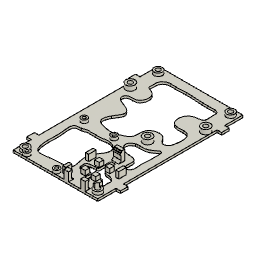
data-logger-inside-frame-504040 v42 (Autodesk Fusion 360 design; units mm, degrees)
Autodesk Fusion 360 part; units mm, degrees
sketch "Sketch1" plane through (0, 0, 0) normal (0, 0, 1) x (1, 0, 0)
  circle A0 centre (0, 0) radius 1.5
  circle A1 centre (0, 88) radius 1.5
  circle A2 centre (48, 0) radius 1.5
  circle A3 centre (48, 88) radius 1.5
  line L0 (-4, 92) -> (52, 92)
  line L1 (52, 92) -> (52, -4)
  line L2 (52, -4) -> (-4, -4)
  line L3 (-4, -4) -> (-4, 92)
  line L4 (-4, 80) -> (-7, 80)
  line L5 (-7, 80) -> (-7, 75)
  line L6 (-7, 75) -> (-4, 75)
  line L7 (-4, 75) -> (-4, 80)
  line L8 (52, 80) -> (55, 80)
  line L9 (55, 80) -> (55, 75)
  line L10 (55, 75) -> (52, 75)
  line L11 (52, 75) -> (52, 80)
  line L12 (-4, 13) -> (-7, 13)
  line L13 (-7, 13) -> (-7, 8)
  line L14 (-7, 8) -> (-4, 8)
  line L15 (-4, 8) -> (-4, 13)
  line L16 (52, 8) -> (55, 8)
  line L17 (55, 8) -> (55, 13)
  line L18 (55, 13) -> (52, 13)
  line L19 (52, 13) -> (52, 8)
  dimension "d1" = 3
  dimension "d2" = 3
  dimension "d3" = 88
  dimension "d4" = 3
  dimension "d5" = 48
  dimension "d6" = 3
  dimension "d7" = 56
  dimension "d8" = 96
  dimension "d9" = 4
  dimension "d10" = 4
  dimension "d11" = 3
  dimension "d12" = 5
  dimension "d13" = 3
  dimension "d14" = 5
  dimension "d15" = 3
  dimension "d16" = 5
  dimension "d17" = 3
  dimension "d18" = 5
  dimension "d19" = 12
  dimension "d20" = 12
  dimension "d21" = 12
  dimension "d22" = 12
  constraint coincident A0.centre origin
  constraint horizontal L0
  constraint vertical L1
  constraint horizontal L2
  constraint vertical L3
  constraint vertical A0.centre A1.centre
  constraint horizontal A0.centre A2.centre
  constraint horizontal A1.centre A3.centre
  constraint horizontal L4
  constraint vertical L5
  constraint horizontal L6
  constraint vertical L7
  constraint coincident L3 L4.start
  constraint horizontal L8
  constraint vertical L9
  constraint horizontal L10
  constraint vertical L11
  constraint coincident L1 L8.start
  constraint horizontal L12
  constraint vertical L13
  constraint horizontal L14
  constraint vertical L15
  constraint coincident L3 L12.start
  constraint horizontal L16
  constraint vertical L17
  constraint horizontal L18
  constraint vertical L19
  constraint coincident L1 L16.start
  measures "d1" diameter of A0
  measures "d2" diameter of A1
  measures "d3" distance of A0.centre A1.centre
  measures "d4" diameter of A2
  measures "d5" distance of A0.centre A2.centre
  measures "d6" diameter of A3
  measures "d7" distance of L0.start L0.end
  measures "d8" distance of L0.start L2.end
  measures "d9" distance of A1.centre L0
  measures "d10" distance of A1.centre L3
  measures "d11" distance of L4.start L4.end
  measures "d12" distance of L4.start L6.end
  measures "d13" distance of L8.start L8.end
  measures "d14" distance of L8.start L10.end
  measures "d15" distance of L12.start L12.end
  measures "d16" distance of L12.start L14.end
  measures "d17" distance of L16.start L16.end
  measures "d18" distance of L16.start L18.end
  measures "d19" distance of L0 L4
  measures "d20" distance of L2 L14
  measures "d21" distance of L2 L16
  measures "d22" distance of L0 L8
extrude "Extrude1" add sketch "Sketch1" along normal blind 1.5
sketch "Sketch2" plane through (0, 0, 1.5) normal (0, 0, 1) x (-1, 0, 0)
  circle A0 centre (-48, -88) radius 1.5
  circle A1 centre (-48, 0) radius 1.5
  circle A2 centre (0, 0) radius 1.5
  circle A3 centre (0, -88) radius 1.5
  line L0 (-52, -8) -> (-55, -8)
  line L1 (-55, -8) -> (-55, -13)
  line L2 (-55, -13) -> (-52, -13)
  line L3 (-52, -13) -> (-52, -75)
  line L4 (-52, -75) -> (-55, -75)
  line L5 (-55, -75) -> (-55, -80)
  line L6 (-55, -80) -> (-52, -80)
  line L7 (-52, -80) -> (-52, -92)
  line L8 (-52, -92) -> (4, -92)
  line L9 (4, -92) -> (4, -80)
  line L10 (4, -80) -> (7, -80)
  line L11 (7, -80) -> (7, -75)
  line L12 (7, -75) -> (4, -75)
  line L13 (4, -75) -> (4, -13)
  line L14 (4, -13) -> (7, -13)
  line L15 (7, -13) -> (7, -8)
  line L16 (7, -8) -> (4, -8)
  line L17 (4, -8) -> (4, 4)
  line L18 (4, 4) -> (-52, 4)
  line L19 (-52, 4) -> (-52, -8)
  line L20 (-27.6361, 2) -> (-45.6361, 2)
  line L21 (-45.6361, 2) -> (-45.6361, -24.25)
  line L22 (-45.6361, -24.25) -> (-27.6361, -24.25)
  line L23 (-27.6361, -24.25) -> (-27.6361, 2)
  line L24 (-29.6361, 2) -> (-32.6361, 2)
  line L25 (-32.6361, 2) -> (-32.6361, 4)
  line L26 (-32.6361, 4) -> (-29.6361, 4)
  line L27 (-29.6361, 4) -> (-29.6361, 2)
  line L28 (-40.6361, 2) -> (-43.6361, 2)
  line L29 (-43.6361, 2) -> (-43.6361, 4)
  line L30 (-43.6361, 4) -> (-40.6361, 4)
  line L31 (-40.6361, 4) -> (-40.6361, 2)
  line L32 (-34.1361, -24.25) -> (-39.1361, -24.25)
  line L33 (-39.1361, -24.25) -> (-39.1361, -26.75)
  line L34 (-39.1361, -26.75) -> (-34.1361, -26.75)
  line L35 (-34.1361, -26.75) -> (-34.1361, -24.25)
  line L36 (-27.6361, -19.25) -> (-25.6361, -19.25)
  line L37 (-25.6361, -19.25) -> (-25.6361, -14.25)
  line L38 (-25.6361, -14.25) -> (-27.6361, -14.25)
  line L39 (-27.6361, -14.25) -> (-27.6361, -19.25)
  line L40 (-45.6361, -19.25) -> (-47.6361, -19.25)
  line L41 (-47.6361, -19.25) -> (-47.6361, -14.25)
  line L42 (-47.6361, -14.25) -> (-45.6361, -14.25)
  line L43 (-45.6361, -14.25) -> (-45.6361, -19.25)
  line L44 (-27.6361, 0.8186) -> (-25.6361, 0.8186)
  line L45 (-25.6361, 0.8186) -> (-25.6361, -3.1814)
  line L46 (-25.6361, -3.1814) -> (-27.6361, -3.1814)
  line L47 (-27.6361, -3.1814) -> (-27.6361, 0.8186)
  line L48 (-45.6361, 0.5806) -> (-47.6361, 0.5806)
  line L49 (-47.6361, 0.5806) -> (-47.6361, -3.4194)
  line L50 (-47.6361, -3.4194) -> (-45.6361, -3.4194)
  line L51 (-45.6361, -3.4194) -> (-45.6361, 0.5806)
  line L52 (-0.7361, -38.1) -> (-24.9361, -38.1)
  line L53 (-24.9361, -38.1) -> (-24.9361, 4)
  line L54 (-24.9361, 4) -> (-0.7361, 4)
  line L55 (-0.7361, 4) -> (-0.7361, -38.1)
  circle A4 centre (-2.9611, -36.05) radius 1
  circle A5 centre (-2.9611, 1.95) radius 1
  circle A6 centre (-22.7111, -36.05) radius 1
  circle A7 centre (-22.7111, 1.95) radius 1
  circle A8 centre (-2.9611, -36.05) radius 2.05
  circle A9 centre (-22.7111, -36.05) radius 2.05
  circle A10 centre (-2.9611, 1.95) radius 2.05
  circle A11 centre (-22.7111, 1.95) radius 2.05
  circle A12 centre (0, 0) radius 2.75
  circle A13 centre (-48, 0) radius 2.75
  circle A14 centre (0, -88) radius 2.75
  circle A15 centre (-48, -88) radius 2.75
  circle A16 centre (1, -70.5) radius 3
  circle A17 centre (-49, -70.5) radius 3
  circle A18 centre (-35.5, -45.5) radius 3
  line L56 (-51.3515, -29.8744) -> (-23.0253, -29.8744)
  line L57 (-23.0253, -29.8744) -> (-23.0253, 4)
  line L58 (-23.0253, 4) -> (-51.3515, 4)
  line L59 (-51.3515, 4) -> (-51.3515, -29.8744)
  dimension "d25" = 18
  dimension "d26" = 26.25
  dimension "d27" = 2
  dimension "d28" = 3
  dimension "d29" = 3
  dimension "d30" = 2
  dimension "d31" = 2
  dimension "d32" = 5
  dimension "d33" = 2.5
  dimension "d34" = 6.5
  dimension "d35" = 2
  dimension "d36" = 5
  dimension "d37" = 2
  dimension "d38" = 5
  dimension "d39" = 5
  dimension "d40" = 5
  dimension "d41" = 2
  dimension "d42" = 4
  dimension "d43" = 2
  dimension "d44" = 4
  dimension "d45" = 42.1
  dimension "d46" = 24.2
  dimension "d47" = 2
  dimension "d48" = 2
  dimension "d49" = 2
  dimension "d50" = 2
  dimension "d51" = 19.75
  dimension "d52" = 38
  dimension "d53" = 2.05
  dimension "d54" = 2.225
  dimension "d57" = 0.7
  dimension "d76" = 5.5
  dimension "d77" = 5.5
  dimension "d78" = 5.5
  dimension "d79" = 5.5
  dimension "d141" = 6
  dimension "d142" = 6
  dimension "d143" = 6
  dimension "d144" = 50
  dimension "d145" = 25
  dimension "d146" = 13.5
  dimension "d149" = 21.5
  dimension "d150" = 7.4
  constraint horizontal L20
  constraint vertical L21
  constraint horizontal L22
  constraint vertical L23
  constraint horizontal L24
  constraint vertical L25
  constraint horizontal L26
  constraint vertical L27
  constraint coincident L20 L24.start
  constraint horizontal L28
  constraint vertical L29
  constraint horizontal L30
  constraint vertical L31
  constraint coincident L20 L28.start
  constraint horizontal L32
  constraint vertical L33
  constraint horizontal L34
  constraint vertical L35
  constraint coincident L22 L32.start
  constraint horizontal L36
  constraint vertical L37
  constraint horizontal L38
  constraint vertical L39
  constraint coincident L23 L36.start
  constraint horizontal L40
  constraint vertical L41
  constraint horizontal L42
  constraint vertical L43
  constraint coincident L21 L40.start
  constraint horizontal L44
  constraint vertical L45
  constraint horizontal L46
  constraint vertical L47
  constraint coincident L23 L44.start
  constraint horizontal L48
  constraint vertical L49
  constraint horizontal L50
  constraint vertical L51
  constraint coincident L21 L48.start
  constraint horizontal L52
  constraint vertical L53
  constraint horizontal L54
  constraint vertical L55
  constraint coincident L18 L54.end
  constraint horizontal A4.centre A6.centre
  constraint vertical A4.centre A5.centre
  constraint vertical A6.centre A7.centre
  constraint horizontal A5.centre A7.centre
  constraint concentric A4 A8
  constraint tangent L52 A8
  constraint concentric A6 A9
  constraint tangent L52 A9
  constraint concentric A5 A10
  constraint tangent L54 A10
  constraint concentric A7 A11
  constraint tangent L54 A11
  constraint coincident A2.centre A12.centre
  constraint concentric A1 A13
  constraint concentric A3 A14
  constraint concentric A0 A15
  constraint horizontal A16.centre A17.centre
  constraint tangent L3 A17
  constraint horizontal L56
  constraint vertical L57
  constraint horizontal L58
  constraint vertical L59
  constraint coincident L54 L57.end
  measures "d25" distance of L20.start L20.end
  measures "d26" distance of L20.start L22.end
  measures "d27" distance of L18 L20
  measures "d28" distance of L24.start L24.end
  measures "d29" distance of L28.start L28.end
  measures "d30" distance of L23 L26.end
  measures "d31" distance of L21 L29
  measures "d32" distance of L32.start L32.end
  measures "d33" distance of L32.start L34.end
  measures "d34" distance of L21 L33
  measures "d35" distance of L36.start L36.end
  measures "d36" distance of L36.start L38.end
  measures "d37" distance of L40.start L40.end
  measures "d38" distance of L40.start L42.end
  measures "d39" distance of L22 L36
  measures "d40" distance of L22 L40
  measures "d41" distance of L44.start L44.end
  measures "d42" distance of L44.start L46.end
  measures "d43" distance of L48.start L48.end
  measures "d44" distance of L48.start L50.end
  measures "d45" distance of L52.start L54.end
  measures "d46" distance of L52.start L52.end
  measures "d47" diameter of A4
  measures "d48" diameter of A5
  measures "d49" diameter of A6
  measures "d50" diameter of A7
  measures "d51" distance of A4.centre A6.centre
  measures "d52" distance of A4.centre A5.centre
  measures "d53" distance of L52 A4.centre
  measures "d54" distance of L55 A4.centre
  measures "d57" distance of L37 L53
  measures "d76" diameter of A12
  measures "d77" diameter of A13
  measures "d78" diameter of A14
  measures "d79" diameter of A15
  measures "d141" diameter of A16
  measures "d142" diameter of A17
  measures "d143" diameter of A18
  measures "d144" distance of A16.centre A17.centre
  measures "d145" vertical distance of A16.centre A18.centre
  measures "d146" horizontal distance of A17.centre A18.centre
  measures "d149" distance of L8 A16.centre
  measures "d150" distance of L52 A18.centre
extrude "Extrude21" add sketch "Sketch2" along normal blind 3 contours A17 | A16 | A18
extrude "Extrude6" add sketch "Sketch2" along normal blind 2 contours A1 L21 L48 L49 A13 | L21 L51 A13 | A2 L55 A10 A12 | A2 L55 A10 A12 | A2 L55 A12 | A14 | A15
extrude "Extrude3" cut sketch "Sketch2" against normal blind 3 contours A7 L57 | A7 L57 | A5 A12 | A5 A12 | A4 | A6
extrude "Extrude2" add sketch "Sketch2" along normal blind 2 contours A9 | A8 | A7 A11 L57 | A7 A11 L57 | A5 A10 A12 | A2 A5 A10 A12 | A2 A10
sketch "Sketch3" plane through (0, 0, 1.5) normal (0, 0, 1) x (-1, 0, 0)
  line L0 (-41.6361, -5) -> (-38.6361, -5)
  line L1 (-38.6361, -5) -> (-38.6361, -8)
  line L2 (-38.6361, -8) -> (-41.6361, -8)
  line L3 (-41.6361, -8) -> (-41.6361, -5)
  line L4 (-34.6361, -5) -> (-31.6361, -5)
  line L5 (-31.6361, -5) -> (-31.6361, -8)
  line L6 (-31.6361, -8) -> (-34.6361, -8)
  line L7 (-34.6361, -8) -> (-34.6361, -5)
  line L8 (-41.6361, -14.25) -> (-38.6361, -14.25)
  line L9 (-38.6361, -14.25) -> (-38.6361, -17.25)
  line L10 (-38.6361, -17.25) -> (-41.6361, -17.25)
  line L11 (-41.6361, -17.25) -> (-41.6361, -14.25)
  line L12 (-31.6361, -14.25) -> (-34.6361, -14.25)
  line L13 (-34.6361, -14.25) -> (-34.6361, -17.25)
  line L14 (-34.6361, -17.25) -> (-31.6361, -17.25)
  line L15 (-31.6361, -17.25) -> (-31.6361, -14.25)
  line L16 (-27.6361, 2) -> (-45.6361, 2)
  line L17 (-45.6361, 2) -> (-45.6361, -24.25)
  line L18 (-45.6361, -24.25) -> (-27.6361, -24.25)
  line L19 (-27.6361, -24.25) -> (-27.6361, 2)
  dimension "d60" = 3
  dimension "d61" = 3
  dimension "d62" = 3
  dimension "d63" = 3
  dimension "d64" = 3
  dimension "d65" = 3
  dimension "d66" = 3
  dimension "d67" = 3
  dimension "d68" = 7
  dimension "d69" = 4
  dimension "d70" = 7
  dimension "d71" = 4
  constraint horizontal L0
  constraint vertical L1
  constraint horizontal L2
  constraint vertical L3
  constraint horizontal L4
  constraint vertical L5
  constraint horizontal L6
  constraint vertical L7
  constraint horizontal L8
  constraint vertical L9
  constraint horizontal L10
  constraint vertical L11
  constraint horizontal L12
  constraint vertical L13
  constraint horizontal L14
  constraint vertical L15
  constraint horizontal L0.start L4.start
  constraint vertical L0.start L8.start
  constraint horizontal L8.start L12.end
  constraint vertical L4.start L12.end
  measures "d60" distance of L0.start L0.end
  measures "d61" distance of L0.start L2.end
  measures "d62" distance of L4.start L4.end
  measures "d63" distance of L4.start L6.end
  measures "d64" distance of L8.start L8.end
  measures "d65" distance of L8.start L10.end
  measures "d66" distance of L12.start L12.end
  measures "d67" distance of L12.start L14.end
  measures "d68" distance of L0 L16
  measures "d69" distance of L3 L17
  measures "d70" distance of L10 L18
  measures "d71" distance of L5 L19
extrude "Extrude4" add sketch "Sketch3" along normal blind 3 contours L0 L1 L2 L3 | L4 L5 L6 L7 | L8 L9 L10 L11 | L12 L13 L14 L15
extrude "Extrude5" add sketch "Sketch2" along normal blind 4.2 contours A1 L21 L48 L49 L51 A13 | L21 L49 L50 L51 A13 | L18 L20 L28 L29 L30 L31 L58 | L21 L40 L41 L42 L43 | L18 L20 L24 L25 L26 L27 L58 | L22 L32 L33 L34 L35 | L23 L44 L45 L46 L47 | L23 L36 L37 L38 L39
sketch "Sketch4" plane through (0, 0, 5.7) normal (0, 0, 1) x (-1, 0, 0)
  line L0 (-34.1361, -26.75) -> (-34.1361, -24.25)
  line L1 (-34.1361, -24.25) -> (-39.1361, -24.25)
  line L2 (-39.1361, -24.25) -> (-39.1361, -26.75)
  line L3 (-39.1361, -26.75) -> (-34.1361, -26.75)
  line L4 (-34.1361, -26.75) -> (-39.1361, -26.75)
  line L5 (-39.1361, -26.75) -> (-39.1361, -23.75)
  line L6 (-39.1361, -23.75) -> (-34.1361, -23.75)
  line L7 (-34.1361, -23.75) -> (-34.1361, -26.75)
  dimension "d82" = 5
  dimension "d83" = 3
  constraint horizontal L4
  constraint vertical L5
  constraint horizontal L6
  constraint vertical L7
  constraint coincident L0.start L3.end
  measures "d82" distance of L0.start L2.end
  measures "d83" distance of L0.start L6.end
extrude "Extrude7" add sketch "Sketch4" along normal blind 1.5
sketch "Sketch5" plane through (0, 0, 5.7) normal (0, 0, 1) x (-1, 0, 0)
  line L0 (-27.6361, -14.25) -> (-27.6361, -19.25)
  line L1 (-27.6361, -19.25) -> (-25.6361, -19.25)
  line L2 (-25.6361, -19.25) -> (-25.6361, -14.25)
  line L3 (-25.6361, -14.25) -> (-27.6361, -14.25)
  line L4 (-25.6361, -19.25) -> (-28.1361, -19.25)
  line L5 (-28.1361, -19.25) -> (-28.1361, -14.25)
  line L6 (-28.1361, -14.25) -> (-25.6361, -14.25)
  line L7 (-25.6361, -14.25) -> (-25.6361, -19.25)
  dimension "d86" = 2.5
  dimension "d87" = 5
  constraint horizontal L4
  constraint vertical L5
  constraint horizontal L6
  constraint vertical L7
  constraint coincident L1.end L2.start
  measures "d86" distance of L1.end L4.end
  measures "d87" distance of L1.end L2.end
sketch "Sketch9" plane through (0, 0, 5.7) normal (0, 0, 1) x (-1, 0, 0)
  line L0 (-29.6361, 4) -> (-32.6361, 4)
  line L1 (-32.6361, 4) -> (-32.6361, 2)
  line L2 (-32.6361, 2) -> (-29.6361, 2)
  line L3 (-29.6361, 2) -> (-29.6361, 4)
  line L4 (-29.6361, 4) -> (-32.6361, 4)
  line L5 (-32.6361, 4) -> (-32.6361, 1.5)
  line L6 (-32.6361, 1.5) -> (-29.6361, 1.5)
  line L7 (-29.6361, 1.5) -> (-29.6361, 4)
  dimension "d103" = 2.5
  constraint horizontal L4
  constraint vertical L5
  constraint horizontal L6
  constraint vertical L7
  constraint coincident L0.start L3.end
  constraint coincident L5.end L6.start
  measures "d103" distance of L0.start L6.end
extrude "Extrude12" add sketch "Sketch9" along normal blind 1.5
sketch "Sketch10" plane through (0, 0, 5.7) normal (0, 0, 1) x (-1, 0, 0)
  line L0 (-40.6361, 4) -> (-43.6361, 4)
  line L1 (-43.6361, 4) -> (-43.6361, 2)
  line L2 (-43.6361, 2) -> (-40.6361, 2)
  line L3 (-40.6361, 2) -> (-40.6361, 4)
  line L4 (-40.6361, 4) -> (-43.6361, 4)
  line L5 (-43.6361, 4) -> (-43.6361, 1.5)
  line L6 (-43.6361, 1.5) -> (-40.6361, 1.5)
  line L7 (-40.6361, 1.5) -> (-40.6361, 4)
  dimension "d167" = 2.5
  constraint horizontal L4
  constraint vertical L5
  constraint horizontal L6
  constraint vertical L7
  constraint coincident L0.start L3.end
  measures "d167" distance of L0.start L6.end
extrude "Extrude27" add sketch "Sketch10" along normal blind 1.5
chamfer "Chamfer4" distance 0.5 angle 45 3 edges at (42.1361, -1.5, 5.7) (31.1361, -1.5, 5.7) (36.6361, 23.75, 5.7) measured on face at (42.6361, -1.5, 6.2) measured on face at (31.6361, -1.5, 6.2) measured on face at (37.4695, 23.9167, 5.7)
thread "Thread2" [suppressed]
sketch "Sketch17" plane through (0, 0, 4.5) normal (0, 0, 1) x (-1, 0, 0)
  circle A0 centre (1, -70.5) radius 3
  circle A1 centre (1, -70.5) radius 1.5
  dimension "d153" = 3
  constraint concentric A0 A1
  measures "d153" diameter of A1
extrude "Extrude22" cut sketch "Sketch17" against normal blind 7 contours A1
sketch "Sketch18" plane through (0, 0, 4.5) normal (0, 0, 1) x (-1, 0, 0)
  circle A0 centre (-49, -70.5) radius 3
  circle A1 centre (-49, -70.5) radius 1.5
  dimension "d156" = 3
  constraint concentric A0 A1
  measures "d156" diameter of A1
extrude "Extrude23" cut sketch "Sketch18" against normal blind 7 contours A1
sketch "Sketch19" plane through (0, 0, 4.5) normal (0, 0, 1) x (-1, 0, 0)
  circle A0 centre (-35.5, -45.5) radius 3
  circle A1 centre (-35.5, -45.5) radius 1.5
  dimension "d159" = 3
  constraint concentric A0 A1
  measures "d159" diameter of A1
extrude "Extrude24" cut sketch "Sketch19" against normal blind 7 contours A1
sketch "Sketch20" plane through (0, 0, 1.5) normal (0, 0, 1) x (-1, 0, 0)
  line L0 (-34.1361, -26.75) -> (-39.1361, -26.75)
  line L1 (-39.1361, -26.75) -> (-39.1361, -24.25)
  line L2 (-39.1361, -24.25) -> (-34.1361, -24.25)
  line L3 (-34.1361, -24.25) -> (-34.1361, -26.75)
  line L4 (-43.6361, 2) -> (-43.6361, 4)
  line L5 (-43.6361, 4) -> (-52, 4)
  line L6 (-52, 4) -> (-52, -8)
  line L7 (-52, -13) -> (-52, -70.5)
  circle A0 centre (-49, -70.5) radius 3
  line L8 (-52, -80) -> (-52, -92)
  line L9 (-52, -92) -> (4, -92)
  line L10 (4, -92) -> (4, -80)
  line L11 (4, -75) -> (4, -70.5)
  circle A1 centre (1, -70.5) radius 3
  line L12 (4, -8) -> (4, 4)
  line L13 (4, 4) -> (-2.9611, 4)
  arc A2 (-1.004, 2.5602) -> (-2.9611, 4) centre (-2.9611, 1.95) ccw
  arc A3 (-2.7486, -0.0889) -> (-1.004, 2.5602) centre (0, 0) ccw
  arc A4 (-2.9611, 4) -> (-2.7486, -0.0889) centre (-2.9611, 1.95) ccw
  line L14 (-2.9611, 4) -> (-22.7111, 4)
  circle A5 centre (-22.7111, 1.95) radius 2.05
  line L15 (-22.7111, 4) -> (-29.6361, 4)
  line L16 (-29.6361, 4) -> (-29.6361, 2)
  line L17 (-29.6361, 2) -> (-32.6361, 2)
  line L18 (-32.6361, 2) -> (-32.6361, 4)
  line L19 (-32.6361, 4) -> (-40.6361, 4)
  line L20 (-40.6361, 4) -> (-40.6361, 2)
  line L21 (-40.6361, 2) -> (-43.6361, 2)
  line L22 (-45.6361, -14.25) -> (-45.6361, -19.25)
  line L23 (-45.6361, -19.25) -> (-47.6361, -19.25)
  line L24 (-47.6361, -19.25) -> (-47.6361, -14.25)
  line L25 (-47.6361, -14.25) -> (-45.6361, -14.25)
  line L26 (-27.6361, -14.25) -> (-25.6361, -14.25)
  line L27 (-25.6361, -14.25) -> (-25.6361, -19.25)
  line L28 (-25.6361, -19.25) -> (-27.6361, -19.25)
  line L29 (-27.6361, -19.25) -> (-27.6361, -14.25)
  line L30 (-47.6361, -3.4194) -> (-47.6361, -2.7258)
  arc A6 (-45.6361, -1.4052) -> (-47.6361, -2.7258) centre (-48, 0) ccw
  line L31 (-45.6361, -1.4052) -> (-45.6361, -3.4194)
  line L32 (-45.6361, -3.4194) -> (-47.6361, -3.4194)
  line L33 (-27.6361, -3.1814) -> (-27.6361, 0.8186)
  line L34 (-27.6361, 0.8186) -> (-25.6361, 0.8186)
  line L35 (-25.6361, 0.8186) -> (-25.6361, -3.1814)
  line L36 (-25.6361, -3.1814) -> (-27.6361, -3.1814)
  line L37 (-31.6361, -17.25) -> (-34.6361, -17.25)
  line L38 (-34.6361, -17.25) -> (-34.6361, -14.25)
  line L39 (-34.6361, -14.25) -> (-31.6361, -14.25)
  line L40 (-31.6361, -14.25) -> (-31.6361, -17.25)
  line L41 (-41.6361, -8) -> (-41.6361, -5)
  line L42 (-41.6361, -5) -> (-38.6361, -5)
  line L43 (-38.6361, -5) -> (-38.6361, -8)
  line L44 (-38.6361, -8) -> (-41.6361, -8)
  line L45 (-41.6361, -17.25) -> (-41.6361, -14.25)
  line L46 (-41.6361, -14.25) -> (-38.6361, -14.25)
  line L47 (-38.6361, -14.25) -> (-38.6361, -17.25)
  line L48 (-38.6361, -17.25) -> (-41.6361, -17.25)
  line L49 (-34.6361, -8) -> (-34.6361, -5)
  line L50 (-34.6361, -5) -> (-31.6361, -5)
  line L51 (-31.6361, -5) -> (-31.6361, -8)
  line L52 (-31.6361, -8) -> (-34.6361, -8)
  circle A7 centre (-48, -88) radius 2.75
  circle A8 centre (-35.5, -45.5) radius 3
  circle A9 centre (0, -88) radius 2.75
  circle A10 centre (-22.7111, -36.05) radius 2.05
  circle A11 centre (-2.9611, -36.05) radius 2.05
  spline S0 degree 5 poles (-6, -31) (-6.2089, -31.0339) (-6.6159, -31.1153) (-7.1879, -31.2803) (-7.8646, -31.5655) (-8.5955, -31.9042) (-9.2655, -32.0974) (-9.9265, -32.1123) (-10.6133, -32.0311) (-11.3495, -31.9614) (-12.1493, -31.9557) (-13.0188, -31.9882) (-13.9539, -32.011) (-14.94, -31.9882) (-15.95, -31.9402) (-16.9546, -31.9166) (-17.934, -31.968) (-18.8872, -32.1183) (-19.8451, -32.3353) (-20.8523, -32.5494) (-21.9471, -32.6766) (-23.144, -32.6391) (-24.4104, -32.3902) (-25.6743, -31.9152) (-26.8437, -31.223) (-27.8225, -30.3407) (-28.5269, -29.307) (-28.9041, -28.1664) (-28.9362, -26.9626) (-28.6372, -25.7333) (-28.0528, -24.5033) (-27.2584, -23.2789) (-26.3589, -22.0419) (-25.4727, -20.7585) (-24.7153, -19.3908) (-24.1834, -17.9066) (-23.9382, -16.2903) (-23.99, -14.5526) (-24.2794, -12.7428) (-24.6941, -10.938) (-25.0935, -9.2281) (-25.3296, -7.7021) (-25.2707, -6.4341) (-24.8214, -5.47) (-23.9499, -4.8103) (-22.6896, -4.4111) (-21.1163, -4.2024) (-19.3322, -4.1019) (-17.4465, -4.0304) (-15.559, -3.9263) (-13.739, -3.7625) (-12.0271, -3.5446) (-10.4431, -3.3032) (-8.9917, -3.0875) (-7.6698, -2.9594) (-6.4717, -2.9865) (-5.3975, -3.2362) (-4.4546, -3.7684) (-3.653, -4.6251) (-3.0024, -5.8213) (-2.5079, -7.3358) (-2.1664, -9.1008) (-1.9661, -11.0201) (-1.886, -12.9914) (-1.8959, -14.9248) (-1.9546, -16.7676) (-2.0136, -18.5154) (-2.0062, -20.2553) (-1.8716, -22.1348) (-1.6553, -24.1082) (-1.4471, -26.0598) (-1.3645, -27.8216) (-1.5172, -29.2345) (-1.981, -30.1894) (-2.7647, -30.6805) (-3.7866, -30.8431) (-4.6929, -30.8679) (-5.3624, -30.9117) (-5.7911, -30.9661) (-6, -31) knots 0 0 0 0 0 0 0.01333333 0.02666667 0.04 0.05333333 0.06666667 0.08 0.09333333 0.10666667 0.12 0.13333333 0.14666667 0.16 0.17333333 0.18666667 0.2 0.21333333 0.22666667 0.24 0.25333333 0.26666667 0.28 0.29333333 0.30666667 0.32 0.33333333 0.34666667 0.36 0.37333333 0.38666667 0.4 0.41333333 0.42666667 0.44 0.45333333 0.46666667 0.48 0.49333333 0.50666667 0.52 0.53333333 0.54666667 0.56 0.57333333 0.58666667 0.6 0.61333333 0.62666667 0.64 0.65333333 0.66666667 0.68 0.69333333 0.70666667 0.72 0.73333333 0.74666667 0.76 0.77333333 0.78666667 0.8 0.81333333 0.82666667 0.84 0.85333333 0.86666667 0.88 0.89333333 0.90666667 0.92 0.93333333 0.94666667 0.96 0.97333333 0.98666667 1 1 1 1 1 1
  line L53 (-2, -13) -> (-2, -25)
  spline S1 degree 5 poles (-9, -48) (-8.8705, -47.7679) (-8.6204, -47.2999) (-8.278, -46.5889) (-7.9088, -45.6366) (-7.6339, -44.4848) (-7.5713, -43.4202) (-7.7301, -42.4853) (-8.1022, -41.7096) (-8.66, -41.0988) (-9.3587, -40.633) (-10.1476, -40.2784) (-10.9795, -39.996) (-11.8209, -39.7518) (-12.6619, -39.5263) (-13.5087, -39.3127) (-14.3753, -39.1138) (-15.2765, -38.9403) (-16.2184, -38.8078) (-17.1945, -38.7345) (-18.1912, -38.7375) (-19.1923, -38.8301) (-20.1829, -39.0182) (-21.1544, -39.2968) (-22.1079, -39.6485) (-23.0473, -40.0505) (-23.9745, -40.4818) (-24.8835, -40.9298) (-25.756, -41.3964) (-26.5536, -41.9069) (-27.23, -42.4996) (-27.7445, -43.2139) (-28.0753, -44.0788) (-28.2335, -45.1008) (-28.2739, -46.254) (-28.2775, -47.4907) (-28.3368, -48.7493) (-28.5402, -49.964) (-28.9567, -51.073) (-29.6203, -52.028) (-30.5152, -52.8023) (-31.5902, -53.386) (-32.7718, -53.7808) (-33.9788, -53.9949) (-35.135, -54.0382) (-36.1836, -53.917) (-37.0999, -53.6301) (-37.8838, -53.1777) (-38.5557, -52.5699) (-39.1501, -51.8348) (-39.7106, -51.0281) (-40.2836, -50.2366) (-40.9091, -49.5564) (-41.6111, -49.075) (-42.3898, -48.8539) (-43.2093, -48.9063) (-44.0035, -49.1963) (-44.7019, -49.6614) (-45.248, -50.2279) (-45.625, -50.8301) (-45.8615, -51.4229) (-46.0055, -51.9844) (-46.1082, -52.5204) (-46.2019, -53.0696) (-46.3025, -53.6847) (-46.4112, -54.4132) (-46.5166, -55.2761) (-46.5974, -56.2675) (-46.6258, -57.3604) (-46.5702, -58.5109) (-46.3988, -59.663) (-46.0823, -60.7522) (-45.5969, -61.7131) (-44.927, -62.4891) (-44.0678, -63.0416) (-43.0277, -63.3587) (-41.8319, -63.4664) (-40.5226, -63.4317) (-39.1535, -63.3455) (-37.7852, -63.3095) (-36.4802, -63.4218) (-35.298, -63.7625) (-34.2903, -64.3802) (-33.4954, -65.2753) (-32.9381, -66.4039) (-32.6308, -67.6938) (-32.5753, -69.0557) (-32.7637, -70.3964) (-33.18, -71.6313) (-33.8014, -72.6986) (-34.5989, -73.5643) (-35.5376, -74.2188) (-36.5767, -74.6743) (-37.6698, -74.9631) (-38.7652, -75.1345) (-39.8053, -75.2537) (-40.7323, -75.3926) (-41.4969, -75.6172) (-42.0659, -75.9758) (-42.4302, -76.4876) (-42.6127, -77.1306) (-42.657, -77.8626) (-42.6168, -78.6393) (-42.5446, -79.437) (-42.4834, -80.2562) (-42.4598, -81.104) (-42.4775, -81.9817) (-42.51, -82.8704) (-42.4956, -83.7197) (-42.3613, -84.468) (-42.0427, -85.0599) (-41.5061, -85.4644) (-40.7685, -85.6924) (-39.8793, -85.7819) (-38.9012, -85.7838) (-37.8934, -85.7483) (-36.8899, -85.7086) (-35.9019, -85.6817) (-34.925, -85.6737) (-33.9452, -85.6832) (-32.9452, -85.7057) (-31.9114, -85.7384) (-30.8365, -85.7811) (-29.7178, -85.8346) (-28.5573, -85.8996) (-27.3606, -85.9751) (-26.1368, -86.0577) (-24.8971, -86.14) (-23.6545, -86.2112) (-22.4223, -86.2607) (-21.2125, -86.2791) (-20.0347, -86.2614) (-18.8949, -86.2084) (-17.7939, -86.1302) (-16.7272, -86.0451) (-15.6879, -85.9745) (-14.6684, -85.9369) (-13.6637, -85.9433) (-12.6725, -85.9916) (-11.7009, -86.0608) (-10.7601, -86.1165) (-9.8627, -86.1197) (-9.0205, -86.0346) (-8.2417, -85.8365) (-7.5271, -85.5199) (-6.876, -85.0938) (-6.2907, -84.5763) (-5.7824, -83.989) (-5.3767, -83.3518) (-5.1009, -82.6805) (-4.9673, -81.9856) (-4.9576, -81.2706) (-5.0076, -80.5302) (-5.043, -79.7605) (-5.0121, -78.9686) (-4.9214, -78.182) (-4.8674, -77.4581) (-4.9796, -76.854) (-5.3714, -76.4011) (-6.0767, -76.0704) (-7.0357, -75.7718) (-8.1333, -75.3901) (-9.2245, -74.8118) (-10.1645, -73.9549) (-10.8376, -72.7993) (-11.1832, -71.4111) (-11.1836, -69.9109) (-10.8559, -68.4466) (-10.2424, -67.166) (-9.4016, -66.1871) (-8.399, -65.5737) (-7.2968, -65.2994) (-6.1516, -65.2587) (-5.0173, -65.3066) (-3.9458, -65.289) (-2.9892, -65.0779) (-2.2011, -64.6028) (-1.6389, -63.8866) (-1.3547, -63.0128) (-1.3873, -62.0904) (-1.754, -61.2226) (-2.4403, -60.4666) (-3.402, -59.8313) (-4.5737, -59.2939) (-5.8753, -58.8106) (-7.2199, -58.3297) (-8.5203, -57.8032) (-9.6968, -57.2006) (-10.6825, -56.5151) (-11.4257, -55.7536) (-11.8923, -54.9314) (-12.0683, -54.0652) (-11.9629, -53.1666) (-11.6107, -52.2347) (-11.066, -51.2612) (-10.3962, -50.236) (-9.8195, -49.3686) (-9.3973, -48.6923) (-9.1295, -48.2321) (-9, -48) knots 0 0 0 0 0 0 0.00512821 0.01025641 0.01538462 0.02051282 0.02564103 0.03076923 0.03589744 0.04102564 0.04615385 0.05128205 0.05641026 0.06153846 0.06666667 0.07179487 0.07692308 0.08205128 0.08717949 0.09230769 0.0974359 0.1025641 0.10769231 0.11282051 0.11794872 0.12307692 0.12820513 0.13333333 0.13846154 0.14358974 0.14871795 0.15384615 0.15897436 0.16410256 0.16923077 0.17435897 0.17948718 0.18461538 0.18974359 0.19487179 0.2 0.20512821 0.21025641 0.21538462 0.22051282 0.22564103 0.23076923 0.23589744 0.24102564 0.24615385 0.25128205 0.25641026 0.26153846 0.26666667 0.27179487 0.27692308 0.28205128 0.28717949 0.29230769 0.2974359 0.3025641 0.30769231 0.31282051 0.31794872 0.32307692 0.32820513 0.33333333 0.33846154 0.34358974 0.34871795 0.35384615 0.35897436 0.36410256 0.36923077 0.37435897 0.37948718 0.38461538 0.38974359 0.39487179 0.4 0.40512821 0.41025641 0.41538462 0.42051282 0.42564103 0.43076923 0.43589744 0.44102564 0.44615385 0.45128205 0.45641026 0.46153846 0.46666667 0.47179487 0.47692308 0.48205128 0.48717949 0.49230769 0.4974359 0.5025641 0.50769231 0.51282051 0.51794872 0.52307692 0.52820513 0.53333333 0.53846154 0.54358974 0.54871795 0.55384615 0.55897436 0.56410256 0.56923077 0.57435897 0.57948718 0.58461538 0.58974359 0.59487179 0.6 0.60512821 0.61025641 0.61538462 0.62051282 0.62564103 0.63076923 0.63589744 0.64102564 0.64615385 0.65128205 0.65641026 0.66153846 0.66666667 0.67179487 0.67692308 0.68205128 0.68717949 0.69230769 0.6974359 0.7025641 0.70769231 0.71282051 0.71794872 0.72307692 0.72820513 0.73333333 0.73846154 0.74358974 0.74871795 0.75384615 0.75897436 0.76410256 0.76923077 0.77435897 0.77948718 0.78461538 0.78974359 0.79487179 0.8 0.80512821 0.81025641 0.81538462 0.82051282 0.82564103 0.83076923 0.83589744 0.84102564 0.84615385 0.85128205 0.85641026 0.86153846 0.86666667 0.87179487 0.87692308 0.88205128 0.88717949 0.89230769 0.8974359 0.9025641 0.90769231 0.91282051 0.91794872 0.92307692 0.92820513 0.93333333 0.93846154 0.94358974 0.94871795 0.95384615 0.95897436 0.96410256 0.96923077 0.97435897 0.97948718 0.98461538 0.98974359 0.99487179 1 1 1 1 1 1
  spline S2 degree 5 poles (-33, -40) (-33.2119, -40.0581) (-33.6455, -40.1549) (-34.3207, -40.2449) (-35.2547, -40.2742) (-36.4497, -40.2374) (-37.6509, -40.2175) (-38.8425, -40.3015) (-40.0109, -40.5571) (-41.1431, -41.0173) (-42.2234, -41.6634) (-43.2318, -42.4127) (-44.1469, -43.1465) (-44.9482, -43.7348) (-45.6198, -44.0621) (-46.1519, -44.0518) (-46.5449, -43.6947) (-46.8103, -43.0626) (-46.9675, -42.2649) (-47.0409, -41.4173) (-47.0574, -40.6007) (-47.0429, -39.8414) (-47.0201, -39.1323) (-47.0054, -38.4468) (-47.0067, -37.7543) (-47.0191, -37.0373) (-47.0302, -36.291) (-47.0253, -35.5189) (-46.9928, -34.7299) (-46.9309, -33.9344) (-46.8495, -33.1416) (-46.7651, -32.3587) (-46.696, -31.5885) (-46.6588, -30.8288) (-46.6626, -30.0698) (-46.7076, -29.297) (-46.7848, -28.4964) (-46.8747, -27.6596) (-46.9472, -26.7882) (-46.9602, -25.8997) (-46.8683, -25.0242) (-46.6339, -24.2006) (-46.2368, -23.4729) (-45.6841, -22.8863) (-45.0223, -22.4836) (-44.3225, -22.3006) (-43.6629, -22.3605) (-43.1124, -22.6696) (-42.7122, -23.2109) (-42.4746, -23.9485) (-42.3864, -24.833) (-42.4115, -25.8078) (-42.4923, -26.8141) (-42.5562, -27.7962) (-42.5287, -28.7041) (-42.3457, -29.4973) (-41.9647, -30.1476) (-41.3788, -30.6426) (-40.6241, -30.9886) (-39.7599, -31.2054) (-38.8532, -31.3233) (-37.9613, -31.3792) (-37.1133, -31.4125) (-36.3005, -31.462) (-35.4963, -31.5645) (-34.6696, -31.752) (-33.8, -32.0505) (-32.8949, -32.4778) (-31.999, -33.0417) (-31.1781, -33.7393) (-30.5077, -34.5565) (-30.0586, -35.4667) (-29.8857, -36.4307) (-30.012, -37.3946) (-30.4257, -38.2942) (-31.0917, -39.0667) (-31.7866, -39.5424) (-32.374, -39.8064) (-32.7881, -39.9419) (-33, -40) knots 0 0 0 0 0 0 0.01333333 0.02666667 0.04 0.05333333 0.06666667 0.08 0.09333333 0.10666667 0.12 0.13333333 0.14666667 0.16 0.17333333 0.18666667 0.2 0.21333333 0.22666667 0.24 0.25333333 0.26666667 0.28 0.29333333 0.30666667 0.32 0.33333333 0.34666667 0.36 0.37333333 0.38666667 0.4 0.41333333 0.42666667 0.44 0.45333333 0.46666667 0.48 0.49333333 0.50666667 0.52 0.53333333 0.54666667 0.56 0.57333333 0.58666667 0.6 0.61333333 0.62666667 0.64 0.65333333 0.66666667 0.68 0.69333333 0.70666667 0.72 0.73333333 0.74666667 0.76 0.77333333 0.78666667 0.8 0.81333333 0.82666667 0.84 0.85333333 0.86666667 0.88 0.89333333 0.90666667 0.92 0.93333333 0.94666667 0.96 0.97333333 0.98666667 1 1 1 1 1 1
  spline S3 degree 5 poles (-33.7598, -13.3699) (-33.8766, -13.3699) (-34.1037, -13.3725) (-34.4133, -13.3874) (-34.7212, -13.4429) (-34.9322, -13.59) (-35.006, -13.825) (-35.006, -14.1471) (-34.9823, -14.5463) (-34.9625, -15.0044) (-34.9583, -15.499) (-34.9694, -16.006) (-34.9879, -16.5036) (-35.0028, -16.9752) (-35.0043, -17.4124) (-34.9884, -17.8187) (-34.956, -18.2056) (-34.9125, -18.5878) (-34.866, -18.9791) (-34.8269, -19.3876) (-34.807, -19.8114) (-34.8181, -20.2347) (-34.8712, -20.6344) (-34.9756, -20.9858) (-35.1374, -21.2684) (-35.3589, -21.4715) (-35.6372, -21.6018) (-35.9642, -21.6783) (-36.3269, -21.7237) (-36.708, -21.7563) (-37.0858, -21.7822) (-37.4349, -21.7862) (-37.7299, -21.74) (-37.9506, -21.614) (-38.0861, -21.3858) (-38.1406, -21.0535) (-38.1323, -20.6355) (-38.0873, -20.1621) (-38.0338, -19.6689) (-37.997, -19.1895) (-37.9939, -18.7493) (-38.0263, -18.3566) (-38.0824, -18.0032) (-38.1434, -17.6718) (-38.1902, -17.3412) (-38.2086, -16.9927) (-38.1966, -16.6164) (-38.1676, -16.215) (-38.1436, -15.7993) (-38.1497, -15.3848) (-38.2083, -14.9884) (-38.3339, -14.6248) (-38.5264, -14.3029) (-38.7718, -14.0246) (-39.0502, -13.7882) (-39.3408, -13.5891) (-39.6283, -13.422) (-39.9101, -13.2831) (-40.1969, -13.1704) (-40.5053, -13.082) (-40.8522, -13.0155) (-41.2492, -12.9662) (-41.6947, -12.9263) (-42.1757, -12.8852) (-42.6718, -12.8313) (-43.1597, -12.7542) (-43.6174, -12.6457) (-44.0282, -12.5021) (-44.3847, -12.3255) (-44.6931, -12.1256) (-44.9676, -11.9156) (-45.2251, -11.7082) (-45.4796, -11.5119) (-45.7375, -11.327) (-45.9914, -11.1413) (-46.2253, -10.936) (-46.4206, -10.6919) (-46.5606, -10.3957) (-46.638, -10.0469) (-46.6564, -9.6601) (-46.6274, -9.2574) (-46.5681, -8.8621) (-46.4981, -8.4932) (-46.4369, -8.1587) (-46.4015, -7.8497) (-46.4033, -7.5482) (-46.4458, -7.2347) (-46.5217, -6.8961) (-46.6096, -6.5347) (-46.6749, -6.1715) (-46.679, -5.8359) (-46.589, -5.5589) (-46.385, -5.3647) (-46.0715, -5.2617) (-45.6747, -5.243) (-45.2333, -5.2932) (-44.7905, -5.3943) (-44.3863, -5.5305) (-44.0489, -5.6951) (-43.7886, -5.8929) (-43.6026, -6.1335) (-43.4775, -6.4246) (-43.3922, -6.7671) (-43.3213, -7.1465) (-43.2382, -7.5348) (-43.1187, -7.8985) (-42.9446, -8.2052) (-42.7071, -8.43) (-42.4108, -8.5638) (-42.0744, -8.616) (-41.7223, -8.6069) (-41.3774, -8.5628) (-41.0551, -8.5097) (-40.7538, -8.467) (-40.4578, -8.4456) (-40.1472, -8.4485) (-39.806, -8.4717) (-39.4306, -8.5039) (-39.0385, -8.5277) (-38.6599, -8.5227) (-38.3281, -8.4703) (-38.0709, -8.3574) (-37.9016, -8.1803) (-37.8094, -7.9492) (-37.77, -7.6814) (-37.7553, -7.3962) (-37.744, -7.1078) (-37.7284, -6.8215) (-37.709, -6.538) (-37.691, -6.2558) (-37.6808, -5.9743) (-37.6821, -5.6969) (-37.6968, -5.4271) (-37.726, -5.1667) (-37.77, -4.9117) (-37.8293, -4.6509) (-37.9028, -4.3708) (-37.9863, -4.0614) (-38.0705, -3.7209) (-38.1398, -3.3626) (-38.1746, -3.0093) (-38.1556, -2.6873) (-38.0674, -2.4199) (-37.9021, -2.2211) (-37.663, -2.0899) (-37.3617, -2.017) (-37.0166, -1.9906) (-36.6503, -2.0025) (-36.2879, -2.054) (-35.954, -2.1525) (-35.6697, -2.3072) (-35.4504, -2.5252) (-35.3022, -2.8076) (-35.2202, -3.1461) (-35.1926, -3.5267) (-35.2035, -3.9313) (-35.2371, -4.3412) (-35.2805, -4.7393) (-35.3274, -5.1129) (-35.3762, -5.454) (-35.4276, -5.7594) (-35.4823, -6.0314) (-35.5385, -6.2773) (-35.59, -6.5106) (-35.628, -6.7458) (-35.6426, -6.9946) (-35.6255, -7.2608) (-35.5707, -7.5388) (-35.4751, -7.817) (-35.3383, -8.0815) (-35.1634, -8.3192) (-34.9568, -8.5206) (-34.725, -8.6802) (-34.4733, -8.7969) (-34.2026, -8.875) (-33.9086, -8.9243) (-33.5849, -8.9566) (-33.2275, -8.9832) (-32.8374, -9.0119) (-32.4253, -9.0432) (-32.012, -9.07) (-31.6204, -9.0812) (-31.2709, -9.0642) (-30.9752, -9.0079) (-30.7302, -8.9057) (-30.5129, -8.7583) (-30.2914, -8.5729) (-30.0358, -8.363) (-29.7278, -8.1474) (-29.3739, -7.9506) (-29.0002, -7.7994) (-28.6413, -7.7198) (-28.3314, -7.7332) (-28.095, -7.8539) (-27.9357, -8.0841) (-27.8387, -8.4156) (-27.7806, -8.8323) (-27.7366, -9.3123) (-27.6881, -9.8312) (-27.6322, -10.3637) (-27.5835, -10.8864) (-27.5662, -11.3779) (-27.6085, -11.8204) (-27.7362, -12.2007) (-27.9667, -12.5109) (-28.3025, -12.7497) (-28.7253, -12.9237) (-29.2028, -13.0446) (-29.6976, -13.1268) (-30.1737, -13.1854) (-30.6058, -13.2331) (-30.9852, -13.2785) (-31.3306, -13.3225) (-31.6835, -13.3599) (-32.0871, -13.3837) (-32.5756, -13.3892) (-33.0344, -13.381) (-33.4028, -13.3725) (-33.643, -13.3699) (-33.7598, -13.3699) knots 0 0 0 0 0 0 0.00465116 0.00930233 0.01395349 0.01860465 0.02325581 0.02790698 0.03255814 0.0372093 0.04186047 0.04651163 0.05116279 0.05581395 0.06046512 0.06511628 0.06976744 0.0744186 0.07906977 0.08372093 0.08837209 0.09302326 0.09767442 0.10232558 0.10697674 0.11162791 0.11627907 0.12093023 0.1255814 0.13023256 0.13488372 0.13953488 0.14418605 0.14883721 0.15348837 0.15813953 0.1627907 0.16744186 0.17209302 0.17674419 0.18139535 0.18604651 0.19069767 0.19534884 0.2 0.20465116 0.20930233 0.21395349 0.21860465 0.22325581 0.22790698 0.23255814 0.2372093 0.24186047 0.24651163 0.25116279 0.25581395 0.26046512 0.26511628 0.26976744 0.2744186 0.27906977 0.28372093 0.28837209 0.29302326 0.29767442 0.30232558 0.30697674 0.31162791 0.31627907 0.32093023 0.3255814 0.33023256 0.33488372 0.33953488 0.34418605 0.34883721 0.35348837 0.35813953 0.3627907 0.36744186 0.37209302 0.37674419 0.38139535 0.38604651 0.39069767 0.39534884 0.4 0.40465116 0.40930233 0.41395349 0.41860465 0.42325581 0.42790698 0.43255814 0.4372093 0.44186047 0.44651163 0.45116279 0.45581395 0.46046512 0.46511628 0.46976744 0.4744186 0.47906977 0.48372093 0.48837209 0.49302326 0.49767442 0.50232558 0.50697674 0.51162791 0.51627907 0.52093023 0.5255814 0.53023256 0.53488372 0.53953488 0.54418605 0.54883721 0.55348837 0.55813953 0.5627907 0.56744186 0.57209302 0.57674419 0.58139535 0.58604651 0.59069767 0.59534884 0.6 0.60465116 0.60930233 0.61395349 0.61860465 0.62325581 0.62790698 0.63255814 0.6372093 0.64186047 0.64651163 0.65116279 0.65581395 0.66046512 0.66511628 0.66976744 0.6744186 0.67906977 0.68372093 0.68837209 0.69302326 0.69767442 0.70232558 0.70697674 0.71162791 0.71627907 0.72093023 0.7255814 0.73023256 0.73488372 0.73953488 0.74418605 0.74883721 0.75348837 0.75813953 0.7627907 0.76744186 0.77209302 0.77674419 0.78139535 0.78604651 0.79069767 0.79534884 0.8 0.80465116 0.80930233 0.81395349 0.81860465 0.82325581 0.82790698 0.83255814 0.8372093 0.84186047 0.84651163 0.85116279 0.85581395 0.86046512 0.86511628 0.86976744 0.8744186 0.87906977 0.88372093 0.88837209 0.89302326 0.89767442 0.90232558 0.90697674 0.91162791 0.91627907 0.92093023 0.9255814 0.93023256 0.93488372 0.93953488 0.94418605 0.94883721 0.95348837 0.95813953 0.9627907 0.96744186 0.97209302 0.97674419 0.98139535 0.98604651 0.99069767 0.99534884 1 1 1 1 1 1
  line L54 (-29.7598, -13.3699) -> (-37.7598, -13.3699)
  line L55 (-52, -8) -> (-55, -8)
  line L56 (-55, -8) -> (-55, -13)
  line L57 (-55, -13) -> (-52, -13)
  line L58 (-52, -70.5) -> (-52, -75)
  line L59 (-52, -75) -> (-55, -75)
  line L60 (-55, -75) -> (-55, -80)
  line L61 (-55, -80) -> (-52, -80)
  line L62 (4, -80) -> (7, -80)
  line L63 (7, -80) -> (7, -75)
  line L64 (7, -75) -> (4, -75)
  line L65 (4, -70.5) -> (4, -13)
  line L66 (4, -13) -> (7, -13)
  line L67 (7, -13) -> (7, -8)
  line L68 (7, -8) -> (4, -8)
  point P0 (-22.2937, -32.6403)
  point P1 (-28, -30)
  point P2 (-27.9689, -24.448)
  point P3 (-24, -16)
  point P4 (-25, -6)
  point P5 (-17, -4)
  point P6 (-7, -3)
  point P7 (-3, -6)
  point P8 (-2, -19)
  point P9 (-2, -30)
  point P10 (-15, -39)
  point P11 (-25, -41)
  point P12 (-28, -44)
  point P13 (-29, -51)
  point P14 (-39, -52)
  point P15 (-45, -50)
  point P16 (-46, -52)
  point P17 (-43.309, -63.2344)
  point P18 (-33, -71)
  point P19 (-42, -76)
  point P20 (-42.4785, -81.8822)
  point P21 (-38.6659, -85.7703)
  point P22 (-27, -86)
  point P23 (-19.301, -86.2232)
  point P24 (-9, -86)
  point P25 (-6.24, -84.4868)
  point P26 (-5, -79)
  point P27 (-5.2208, -76.6351)
  point P28 (-9, -66)
  point P29 (-1.5592, -61.8)
  point P30 (-12, -54)
  point P31 (-41, -41)
  point P32 (-46, -44)
  point P33 (-47.0083, -38.3168)
  point P34 (-46.6868, -31.3077)
  point P35 (-43.5681, -22.4659)
  point P36 (-42.4106, -25.3917)
  point P37 (-42, -30)
  point P38 (-38.2208, -31.3589)
  point P39 (-34, -32)
  point P40 (-30, -36)
  point P41 (-38, -19)
  point P42 (-41, -13)
  point P43 (-45.5, -11.5)
  point P44 (-46.5, -8.5)
  point P45 (-46.5, -5.5)
  point P46 (-37.7274, -5.1843)
  point P47 (-34.5036, -8.7737)
  point P48 (-27.7084, -9.6083)
  point P49 (-14, -32)
  point P50 (-11, -32)
  point P51 (-9, -32)
  point P52 (-18, -32)
  point P53 (-8, -42)
  point P54 (-11, -40)
  point P55 (-8, -58)
  point P56 (-35, -54)
  point P57 (-42, -49)
  point P58 (-46.3289, -53.8728)
  point P59 (-46.4798, -59.0066)
  point P60 (-10, -74)
  point P61 (-3, -65)
  point P62 (-5, -82)
  point P63 (-13.4877, -85.959)
  point P64 (-33.4944, -85.6948)
  point P65 (-42, -85)
  point P66 (-42.6295, -78.2583)
  point P67 (-38, -75)
  point P68 (-35, -64)
  point P69 (-20, -39)
  point P70 (-28.2692, -7.7858)
  point P71 (-28, -12.5)
  point P72 (-30.7692, -13.2531)
  point P73 (-39.5, -13.5)
  point P74 (-35.2084, -21.3138)
  point P75 (-44, -12.5)
  point P76 (-46.5, -10.5)
  point P77 (-46.5, -7)
  point P78 (-44.5, -5.5)
  point P79 (-35, -14)
  point P80 (-35, -17)
  point P81 (-34.8346, -19.3512)
  point P82 (-36.7504, -21.7577)
  point P83 (-38, -21.5)
  point P84 (-38.199, -17.0848)
  point P85 (-38.2691, -14.8419)
  point P86 (-38.093, -8.3417)
  point P87 (-42.7792, -8.3417)
  point P88 (-43.4439, -6.5802)
  point P89 (-37, -2)
  point P90 (-35.6336, -6.9126)
  point P91 (-35.5, -2.5)
  point P92 (-31, -9)
  point P93 (-35.4822, -6.0231)
  point P94 (-35.2413, -4.3559)
  point P95 (-35.3677, -8.0093)
  point P96 (-33, -9)
  point P97 (-29.9503, -8.3084)
  point P98 (-37.7607, -7.4776)
  point P99 (-37.6942, -6.2811)
  point P100 (-38, -4)
  point P101 (-38.0598, -2.459)
  point P102 (-39.788, -8.4746)
  point P103 (-41.2504, -8.5411)
  point P104 (-42.432, -12.8551)
  point P105 (-46.8797, -27.5459)
  point P106 (-46.1402, -23.4305)
  point P107 (-47, -35)
  point P108 (-47.0083, -41.6928)
  constraint midpoint P8 L53
  constraint midpoint S3.start L54
  constraint coincident S3 P104
extrude "Extrude25" cut sketch "Sketch20" against normal blind 3 contours S0 | S1 | S2 | S3 L54 | S3 L54
fillet "Fillet2" radius 1.5 3 edges at (31.1361, -2, 1.5) (42.1361, -2, 1.5) (36.6361, 24.25, 1.5)
sketch "Sketch22" plane through (0, 0, 7.2) normal (0, 0, 1) x (-1, 0, 0)
  line L0 (-34.1361, -23.75) -> (-39.1361, -23.75)
  line L1 (-39.1361, -23.75) -> (-39.1361, -26.75)
  line L2 (-39.1361, -26.75) -> (-34.1361, -26.75)
  line L3 (-34.1361, -26.75) -> (-34.1361, -23.75)
  line L4 (-34.1361, -26.75) -> (-39.1361, -26.75)
  line L5 (-39.1361, -26.75) -> (-39.1361, -24.75)
  line L6 (-39.1361, -24.75) -> (-34.1361, -24.75)
  line L7 (-34.1361, -24.75) -> (-34.1361, -26.75)
  dimension "d173" = 5
  dimension "d174" = 2
  constraint horizontal L4
  constraint vertical L5
  constraint horizontal L6
  constraint vertical L7
  constraint coincident L2.end L3.start
  measures "d173" distance of L2.end L1.end
  measures "d174" distance of L2.end L6.end
extrude "Extrude29" add sketch "Sketch22" along normal blind 1 contours L1 L2 L3 L4 L5 L6 L7
thread "Thread6" [suppressed]
fillet "Fillet3" radius 0.5 1 edges at (36.6361, 24.75, 7.2)
split "Split1" [suppressed]
equation "d13 = d11"
equation "d14 = d12"
equation "d15 = d11"
equation "d16 = d12"
equation "d17 = d11"
equation "d18 = d12"
equation "d20 = d19"
equation "d21 = d19"
equation "d22 = d19"
equation "d29 = d28"
equation "d30 = d31"
equation "d32 = d36"
equation "d34 = ( d25 - 5 mm ) / 2"
equation "d37 = d35"
equation "d38 = d36"
equation "d41 = d35"
equation "d43 = d35"
equation "d44 = d42"
equation "d47 = d48"
equation "d49 = d48"
equation "d50 = d48"
equation "d53 = ( d45 - d52 ) / 2"
equation "d54 = ( d46 - d51 ) / 2"
equation "d60 = d66"
equation "d61 = d66"
equation "d62 = d66"
equation "d63 = d66"
equation "d64 = d66"
equation "d65 = d66"
equation "d67 = d66"
equation "d69 = d71"
equation "d70 = d68"
equation "d74 = 3 mm + 1.2 mm"
equation "d76 = d78"
equation "d77 = d78"
equation "d79 = d78"
